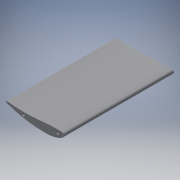
# Autodesk Inventor part: subflap_top
Saved by Autodesk Inventor 2018 (Build 220112000, 112)
## iProperties
Created: 2018-05-24
Part Number: subflap_top
Material: 一般
Document SubType Name: Modeling
Designer: ku_sk
Density: 1 g/cm^3
Appearance: 既定
Author: ku_sk
Autodesk Inventor part; units mm, degrees
ref_plane "YZ Plane" through (0, 0, 0) normal (1, 0, 0) x (0, 1, 0)
ref_plane "XZ Plane" through (0, 0, 0) normal (0, 1, 0) x (-1, 0, 0)
ref_plane "XY Plane" through (0, 0, 0) normal (0, 0, 1) x (1, 0, 0)
sketch "スケッチ1" plane through (0, 0, 0) normal (0, 1, 0) x (-1, 0, 0)
  arc A0 (41.4452, -14.9694) -> (120.7701, -0.6068) centre (36.8758, 236.5065) ccw projected
  arc A1 (30.7183, -14.8468) -> (41.4452, -14.9694) centre (38.1525, 166.2425) ccw projected
  arc A2 (11.0166, -11.3447) -> (30.7183, -14.8468) centre (33.77, 59.49) ccw projected
  arc A3 (-0.3565, -5.7585) -> (11.0166, -11.3447) centre (24.3575, 30.1875) ccw projected
  arc A4 (-3.5852, -2.6234) -> (-0.3565, -5.7585) centre (7.25, 5.305) ccw projected
  arc A5 (-0.7848, 4.3726) -> (-3.5852, -2.6234) centre (0, 0) ccw projected
  arc A6 (7.6183, 5.1344) -> (-0.7848, 4.3726) centre (7.775, -43.32) ccw projected
  arc A7 (35.5607, 3.8888) -> (7.6183, 5.1344) centre (8.565, -287.665) ccw projected
  arc A8 (35.5607, 3.8888) -> (52.6853, 2.3311) centre (526.9475, 5310.875) ccw projected
  arc A9 (52.6853, 2.3311) -> (84.6244, 0.9905) centre (82.86, 340.0849) ccw projected
  arc A10 (84.6244, 0.9905) -> (119.8564, 3.2634) centre (83.0725, 299.245) ccw projected
  arc A11 (120.7701, -0.6068) -> (119.8564, 3.2634) centre (120.103, 1.2786) ccw projected
  point P0 (0, 0)
extrude "押し出し1" add sketch "スケッチ1" along normal mid plane 250
sketch "スケッチ2" plane through (0, -125, 0) normal (0, -1, 0) x (1, 0, 0)
  circle A0 centre (-85, -5) radius 3 projected
  circle A1 centre (-10, -2) radius 3 projected
  point P0 (0, 0)
extrude "押し出し2" cut sketch "スケッチ2" against normal up to next
ref_plane "作業平面2" through (-121.2214, 0, 2.9367) normal (-0.5591926, 0, 0.8290378) x (0, -1, 0)
ref_plane "作業平面1" through (-146.4564, 100, -7.5667) normal (-0.5591926, 0, 0.8290378) x (0.8290378, 0, 0.5591926)
sketch "スケッチ3" plane through (-121.2214, 0, 2.9367) normal (-0.5591926, 0, 0.8290378) x (0, -1, 0)
  arc A0 (-135, -26.7942) -> (-100, 63.2058) centre (-233.2143, 63.2058) ccw projected
  line L0 (-100, 63.2058) -> (-100, 73.2058) projected
  line L1 (-100, 473.2058) -> (-100, 73.2058) projected
  line L2 (-135, -26.7942) -> (-135, 113.2058)
  line L3 (-135, 113.2058) -> (-100, 113.2058)
  point P0 (0, 98.855)
  dimension "d6" = 140
  constraints: 4 end point, 1 perpendicular, 1 point on line, 1 vertical
  measures "d6" distance of L2.start L2.end
extrude "押し出し3" cut sketch "スケッチ3" against normal through all
